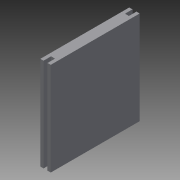
# Autodesk Inventor part: ceiling_case_cover
Saved by Autodesk Inventor 2014 (Build 180170000, 170)
## iProperties
Created: 2014-02-15
Part Number: ceiling_case_cover
Material: Generic
Document SubType Name: Modeling
Designer: anish
Density: 1 g/cm^3
Appearance: Default
Author: anish
Autodesk Inventor part; units mm, degrees
ref_plane "YZ Plane" through (0, 0, 0) normal (1, 0, 0) x (0, 1, 0)
ref_plane "XZ Plane" through (0, 0, 0) normal (0, 1, 0) x (-1, 0, 0)
ref_plane "XY Plane" through (0, 0, 0) normal (0, 0, 1) x (1, 0, 0)
sketch "Sketch1" plane through (0, 0, 0) normal (0, 1, 0) x (-1, 0, 0)
  line L0 (2.8823, 56.4) -> (2.8823, -6.592)
  line L1 (-4.4837, -6.592) -> (-4.4837, 56.4)
  line L2 (0.5963, 56.4) -> (0.5963, 51.066)
  line L3 (0.5963, 51.066) -> (-2.1977, 51.066)
  line L4 (-2.1977, 51.066) -> (-2.1977, 56.4)
  line L5 (0.5963, -6.592) -> (0.5963, -1.258)
  line L6 (0.5963, -1.258) -> (-2.1977, -1.258)
  line L7 (-2.1977, -1.258) -> (-2.1977, -6.592)
  line L8 (-4.4837, 56.4) -> (-2.1977, 56.4)
  line L9 (0.5963, 56.4) -> (2.8823, 56.4)
  line L10 (2.8823, -6.592) -> (0.5963, -6.592)
  line L11 (-2.1977, -6.592) -> (-4.4837, -6.592)
  point P0 (0, 0)
  dimension "d0" = 7.366
  dimension "d1" = 62.992
  dimension "d2" = 2.286
  dimension "d3" = 2.286
  dimension "d5" = 2.286
  dimension "d6" = 2.286
  dimension "d7" = 5.334
  dimension "d8" = 5.334
  dimension "d9" = 5.334
  dimension "d10" = 5.334
  constraints: 24 end point, 7 parallel, 2 horizontal, 2 perpendicular
  measures "d0" distance of L0.end L1.start
  measures "d1" distance of L0.start L0.end
  measures "d2" distance between parallel lines of L0 L2
  measures "d3" distance between parallel lines of L4 L1
  measures "d5" distance between parallel lines of L1 L7
  measures "d6" distance between parallel lines of L0 L5
  measures "d7" distance between parallel lines of L10 L6
  measures "d8" distance between parallel lines of L6 L11
  measures "d9" distance between parallel lines of L3 L8
  measures "d10" distance between parallel lines of L9 L3
extrude "Extrusion1" add sketch "Sketch1" along normal blind 66.04
body "Solid1"
